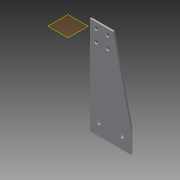
# Autodesk Inventor part: Pneumatic Piston Front Flange (Left Custom)
Saved by Autodesk Inventor 2014 SP1 (Build 180222100, 222)
## iProperties
Created: 2014-01-17
Part Number: Pneumatic Piston Front Flange (Left Custom)
Material: Aluminum 6061
Document SubType Name: Sheet Metal
Designer: Michael
Density: 2.71 g/cm^3
Sheet Metal Rule: Default
Appearance: Aluminum - Flat
Flat Pattern Width: 4.445 cm
Flat Pattern Length: 10.6362 cm
Flat Pattern Area: 47.2781 cm^2
Sheet Metal Width: 1.750 in
Sheet Metal Length: 4.188 in
Sheet Metal Area: 7.328 in^2
Author: Michael
Autodesk Inventor part; units mm, degrees
note: some values were not read from the file. Left out: dimensions or parameters whose unit could not be read.
ref_plane "YZ Plane" through (0, 0, 0) normal (1, 0, 0) x (0, 1, 0)
ref_plane "XZ Plane" through (0, 0, 0) normal (0, 1, 0) x (-1, 0, 0)
ref_plane "XY Plane" through (0, 0, 0) normal (0, 0, 1) x (1, 0, 0)
sketch "Sketch1" plane through (0, 0, 0) normal (0, 0, 1) x (1, 0, 0)
  line L0 (106.3625, -44.45) -> (0, -44.45)
  line L1 (110.551814, -19.05) -> (110.551814, -44.45)
  line L2 (106.3625, -19.05) -> (110.551814, -19.05)
  line L3 (106.3625, -19.05) -> (110.551814, -19.05)
  line L4 (110.551814, -19.05) -> (110.551814, -22.225)
  line L5 (110.551814, -22.225) -> (106.3625, -22.225)
  line L6 (106.3625, -22.225) -> (106.3625, -19.05)
  line L7 (106.3625, -19.05) -> (106.3625, -44.45)
  line L8 (110.551814, -19.05) -> (110.551814, -44.45)
  line L9 (106.3625, -41.275) -> (110.551814, -41.275)
  line L10 (110.551814, -41.275) -> (110.551814, -44.45)
  line L11 (110.551814, -44.45) -> (106.3625, -44.45)
  line L12 (106.3625, -44.45) -> (106.3625, -41.275)
  point P0 (0, 0)
  point P1 (110.551814, -34.925)
  point P2 (111.304505, 0)
  point P3 (131.506814, -44.45)
  point P4 (131.506814, -19.05)
  dimension "d6" = 25.4
  dimension "d22" = 12.7
  dimension "d54" = 25.4
  dimension "d55" = 106.3625
  dimension "d56" = 25.4
  dimension "d57" = 44.45
  dimension "d58" = 9.525
  dimension "d81" = 6.35
  dimension "d82" = 6.35
  dimension "d85" = 12.7
  dimension "d88" = 12.7
  constraints: 12 end point, 6 centre point, 3 horizontal, 2 point on line, 2 vertical, 1 equal radius, 1 parallel, 1 perpendicular, 8 other
  measures "d22" distance between parallel lines of L0 L4
  measures "d54" distance of L0.end L5.end
  measures "d55" distance between parallel lines of L0 L1
  measures "d56" distance of L1.start L1.end
  measures "d57" distance of L0.start L0.end
sketch "Sketch1 outline for Plate1" plane through (0, 0, 0) normal (0, 0, 1) x (1, 0, 0)
  line L0 (0, 106.3625) -> (0, 0)
  line L1 (25.4, 106.3625) -> (0, 106.3625)
  line L2 (0, 0) -> (44.45, 0)
  line L3 (44.45, 25.4) -> (25.4, 106.3625)
  line L4 (44.45, 0) -> (44.45, 25.4)
  circle A0 centre (9.525, 12.7) radius 2.0701
  circle A1 centre (34.925, 12.7) radius 2.0701
  circle A2 centre (6.35, 87.3125) radius 2.0701
  circle A3 centre (6.35, 100.0125) radius 2.0701
  circle A4 centre (19.05, 87.3125) radius 2.0701
  circle A5 centre (19.05, 100.0125) radius 2.0701
extrude "Plate1" add sketch "Sketch1 outline for Plate1" along normal blind 1.5875
ref_plane "Work Plane1" through (0, 110.8075, 25.4) normal (0, 1, 0) x (1, 0, 0)
sketch "Sketch4 outline for Cut3" plane through (0, 110.8075, 25.4) normal (0, 1, 0) x (1, 0, 0)
  line L0 (0, 20.955) -> (0, 0)
  line L1 (0, 0) -> (25.4, 0)
  line L2 (25.4, 0) -> (25.4, 20.955)
  line L3 (25.4, 20.955) -> (0, 20.955)
extrude "Cut3" cut sketch "Sketch4 outline for Cut3" against normal blind 1.5875
fillet "Fillet5" radius 12.7 1 edges at (44.45, 25.4, 0.7937)
sketch "Sketch4" plane through (0, 110.8075, 25.4) normal (0, 1, 0) x (1, 0, 0)
  line L0 (25.4, 0) -> (0, 0)
  circle A0 centre (19.05, 6.35) radius 2.3749
  line L1 (0, 0) -> (0, 20.955)
  line L2 (0, 20.955) -> (25.4, 20.955)
  line L3 (25.4, 20.955) -> (25.4, 21.413463)
  line L4 (21.135301, 0) -> (22.225, 0)
  line L5 (0, 0) -> (0, 20.955)
  line L6 (25.4, 20.955) -> (0, 20.955)
  line L7 (25.4, 20.955) -> (25.4, 17.78)
  line L8 (25.4, 17.78) -> (25.4, 9.525)
  line L9 (12.7, 9.525) -> (12.7, 20.955)
  arc A1 (12.7, 9.525) -> (22.225, 0) centre (22.225, 9.525) ccw
  line L10 (25.4, 20.955) -> (25.4, 0)
  line L11 (0, 0) -> (25.4, 0)
  line L12 (25.4, 0) -> (25.4, 20.955)
  point P0 (0, 25.4)
  point P1 (12.7, 0)
  point P2 (25.4, 0)
  point P3 (12.7, 0)
  dimension "d28" = 4.7498
  dimension "d29" = 6.35
  dimension "d34" = 19.05
  dimension "d47" = 3.175
  dimension "d48" = 6.35
  dimension "d49" = 6.35
  dimension "d50" = 9.525
  constraints: 18 end point, 9 point on line, 3 perpendicular, 2 centre point, 2 midpoint, 2 parallel, 2 point on circle, 2 tangent, 1 collinear, 1 horizontal, 1 vertical
  measures "d28" diameter of A0
  measures "d29" distance from line of L0 A0.centre
  measures "d34" distance from line of L1 A0.centre
  measures "d47" distance of L7.end L6.start
  measures "d48" distance from line of A0.centre L9
  measures "d49" horizontal distance of point (25.4, 0) A0.centre
  measures "d50" radius of A1
equation "\"d51\" = Thickness"
equation "\"BendRadius\" = Thickness"
equation "\"BendReliefWidth\" = Thickness"
equation "\"BendReliefDepth\" = 0.5 * Thickness"
equation "\"CornerReliefSize\" = 4 * Thickness"
equation "\"MinimumRemnant\" = 2 * Thickness"
equation "\"TransitionRadius\" = BendRadius"
equation "\"JacobiRadiusSize\" = BendRadius"
equation "\"GapSize\" = Thickness"
equation "\"d11\" = BendRadius"
equation "\"Thickness\" = 1.5875"
body "Solid1"
